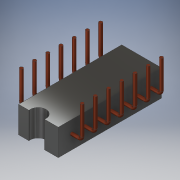
# Autodesk Inventor part: dip7
Saved by Autodesk Inventor 2019 (Build 230136000, 136)
## iProperties
Created: 2020-05-08
Part Number: dip7
Material: Silicon Nitride
Document SubType Name: Modeling
Designer: darkl
Density: 3.18 g/cm^3
Appearance: Chrome - Polished Black
Author: darkl
Autodesk Inventor part; units mm, degrees
ref_plane "YZ Plane" through (0, 0, 0) normal (1, 0, 0) x (0, 1, 0)
ref_plane "XZ Plane" through (0, 0, 0) normal (0, 1, 0) x (-1, 0, 0)
ref_plane "XY Plane" through (0, 0, 0) normal (0, 0, 1) x (1, 0, 0)
sketch "Sketch1" plane through (0, 0, 0) normal (0, 1, 0) x (-1, 0, 0)
  line L0 (4.5856, 19.0159) -> (4.5856, -0.4841)
  line L1 (4.5856, -0.4841) -> (-2.9144, -0.4841)
  line L2 (-2.9144, -0.4841) -> (-2.9144, 19.0159)
  line L3 (-2.9144, 19.0159) -> (4.5856, 19.0159)
  point P0 (0, 0)
  dimension "d0" = 19.5
  dimension "d1" = 7.5
  dimension "d2" = 19.5
  constraints: 8 end point, 2 perpendicular, 1 vertical
  measures "d0" distance of L0.start L0.end
  measures "d1" distance of L0.end L1.end
  measures "d2" distance of L1.end L2.end
extrude "Extrusion1" add sketch "Sketch1" along normal blind 5
sketch "Sketch2" plane through (2.9144, 0, 19.0159) normal (1, 0, 0) x (0, 0, -1)
  circle A0 centre (17.518, 2.6919) radius 0.3
  point P0 (19.0159, 0)
  dimension "d9" = 0.6
  constraints: 1 centre point
  measures "d9" diameter of A0
sketch3d "3D Sketch2"
  line L0 (2.9144, 2.6919, 1.4979) -> (4.3144, 2.6919, 1.4979)
  arc A0 (4.3144, 2.6919, 1.4979) -> (4.9144, 3.2919, 1.4979) centre (4.3144, 3.2919, 1.4979) ccw
  line L1 (4.9144, 3.2919, 1.4979) -> (4.9144, 8.6919, 1.4979)
  dimension "d10" = 2
  dimension "d11" = 6
  dimension "d12" = 0.6
sweep "Sweep1" add profiles "Sketch2" path "3D Sketch2"
sketch "Sketch4" plane through (2.9144, 0, 19.0159) normal (1, 0, 0) x (0, 0, -1)
  circle A0 centre (17.518, 2.6919) radius 0.3 projected
  line L0 (17.518, 2.6919) -> (15.018, 2.6919)
  circle A1 centre (15.018, 2.6919) radius 0.3
  point P0 (19.0159, 0)
  dimension "d15" = 2.5
  dimension "d16" = 0.6
  constraints: 2 end point, 1 centre point, 1 coincident, 1 horizontal
  measures "d15" distance of L0.start L0.end
  measures "d16" diameter of A1
sketch3d "3D Sketch3"
  line L0 (2.9144, 2.6919, 3.9979) -> (4.3144, 2.6919, 3.9979)
  arc A0 (4.3144, 2.6919, 3.9979) -> (4.9144, 3.2919, 3.9979) centre (4.3144, 3.2919, 3.9979) ccw
  line L1 (4.9144, 3.2919, 3.9979) -> (4.9144, 8.6919, 3.9979)
  dimension "d17" = 2
  dimension "d18" = 6
  dimension "d19" = 0.6
sweep "Sweep2" add profiles "Sketch4" path "3D Sketch3" contours A1
sketch "Sketch5" plane through (2.9144, 0, 19.0159) normal (1, 0, 0) x (0, 0, -1)
  circle A0 centre (15.018, 2.6919) radius 0.3 projected
  line L0 (15.018, 2.6919) -> (12.518, 2.6919)
  circle A1 centre (12.518, 2.6919) radius 0.3
  point P0 (19.0159, 0)
  dimension "d22" = 2.5
  dimension "d23" = 0.6
  constraints: 2 end point, 1 centre point, 1 coincident, 1 horizontal
  measures "d22" distance of L0.start L0.end
  measures "d23" diameter of A1
sketch3d "3D Sketch4"
  line L0 (2.9144, 2.6919, 6.4979) -> (4.3144, 2.6919, 6.4979)
  arc A0 (4.3144, 2.6919, 6.4979) -> (4.9144, 3.2919, 6.4979) centre (4.3144, 3.2919, 6.4979) ccw
  line L1 (4.9144, 3.2919, 6.4979) -> (4.9144, 8.6919, 6.4979)
  dimension "d24" = 2
  dimension "d25" = 6
  dimension "d26" = 0.6
sweep "Sweep3" add profiles "Sketch5" path "3D Sketch4" contours A1
sketch "Sketch6" plane through (2.9144, 0, 19.0159) normal (1, 0, 0) x (0, 0, -1)
  circle A0 centre (12.518, 2.6919) radius 0.3 projected
  line L0 (12.518, 2.6919) -> (10.018, 2.6919)
  circle A1 centre (10.018, 2.6919) radius 0.3
  line L1 (10.018, 2.6919) -> (7.518, 2.6919)
  circle A2 centre (7.518, 2.6919) radius 0.3
  line L2 (7.518, 2.6919) -> (5.018, 2.6919)
  circle A3 centre (5.018, 2.6919) radius 0.3
  line L3 (5.018, 2.6919) -> (2.518, 2.6919)
  circle A4 centre (2.518, 2.6919) radius 0.3
  point P0 (19.0159, 0)
  dimension "d29" = 2.5
  dimension "d30" = 0.6
  dimension "d31" = 2.5
  dimension "d32" = 0.6
  dimension "d33" = 2.5
  dimension "d34" = 0.6
  dimension "d35" = 2.5
  dimension "d36" = 0.6
  constraints: 8 end point, 4 centre point, 4 coincident, 3 horizontal, 1 point on line
  measures "d29" distance of L0.start L0.end
  measures "d30" diameter of A1
  measures "d31" distance of L1.start L1.end
  measures "d32" diameter of A2
  measures "d33" distance of L2.start L2.end
  measures "d34" diameter of A3
  measures "d35" distance of L3.start L3.end
  measures "d36" diameter of A4
sketch3d "3D Sketch5"
  line L0 (2.9144, 2.6919, 8.9979) -> (4.3144, 2.6919, 8.9979)
  arc A0 (4.3144, 2.6919, 8.9979) -> (4.9144, 3.2919, 8.9979) centre (4.3144, 3.2919, 8.9979) ccw
  line L1 (4.9144, 3.2919, 8.9979) -> (4.9144, 8.6919, 8.9979)
  dimension "d37" = 2
  dimension "d38" = 6
  dimension "d39" = 0.6
sweep "Sweep4" add profiles "Sketch6" path "3D Sketch5" contours A1 L1 L0 | L0 L1 A1
sketch "Sketch7" plane through (2.9144, 0, 19.0159) normal (1, 0, 0) x (0, 0, -1)
  circle A0 centre (10.018, 2.6919) radius 0.3 projected
  line L0 (10.018, 2.6919) -> (7.518, 2.6919)
  circle A1 centre (7.518, 2.6919) radius 0.3
  point P0 (19.0159, 0)
  dimension "d42" = 2.5
  dimension "d43" = 0.6
  constraints: 2 end point, 1 centre point, 1 coincident, 1 horizontal
  measures "d42" distance of L0.start L0.end
  measures "d43" diameter of A1
sketch3d "3D Sketch7"
  line L0 (2.9144, 2.6919, 11.4979) -> (4.3144, 2.6919, 11.4979)
  arc A0 (4.3144, 2.6919, 11.4979) -> (4.9144, 3.2919, 11.4979) centre (4.3144, 3.2919, 11.4979) ccw
  line L1 (4.9144, 3.2919, 11.4979) -> (4.9144, 8.6919, 11.4979)
  dimension "d44" = 2
  dimension "d45" = 6
  dimension "d46" = 0.6
sweep "Sweep5" add profiles "Sketch7" path "3D Sketch7" contours A1
sketch "Sketch8" plane through (2.9144, 0, 19.0159) normal (1, 0, 0) x (0, 0, -1)
  circle A0 centre (7.518, 2.6919) radius 0.3 projected
  line L0 (7.518, 2.6919) -> (5.018, 2.6919)
  circle A1 centre (5.018, 2.6919) radius 0.3
  point P0 (19.0159, 0)
  dimension "d49" = 2.5
  dimension "d50" = 0.6
  constraints: 2 end point, 1 centre point, 1 coincident, 1 horizontal
  measures "d49" distance of L0.start L0.end
  measures "d50" diameter of A1
sketch3d "3D Sketch9"
  line L0 (2.9144, 2.6919, 13.9979) -> (4.3144, 2.6919, 13.9979)
  arc A0 (4.3144, 2.6919, 13.9979) -> (4.9144, 3.2919, 13.9979) centre (4.3144, 3.2919, 13.9979) ccw
  line L1 (4.9144, 3.2919, 13.9979) -> (4.9144, 8.6919, 13.9979)
  dimension "d51" = 2
  dimension "d52" = 6
  dimension "d53" = 0.6
sweep "Sweep6" add profiles "Sketch8" path "3D Sketch9" contours A1
sketch "Sketch9" plane through (2.9144, 0, 19.0159) normal (1, 0, 0) x (0, 0, -1)
  circle A0 centre (5.018, 2.6919) radius 0.3 projected
  line L0 (5.018, 2.6919) -> (2.518, 2.6919)
  circle A1 centre (2.518, 2.6919) radius 0.3
  point P0 (19.0159, 0)
  dimension "d56" = 2.5
  dimension "d57" = 0.6
  constraints: 2 end point, 1 centre point, 1 coincident, 1 horizontal
  measures "d56" distance of L0.start L0.end
  measures "d57" diameter of A1
sketch3d "3D Sketch10"
  line L0 (2.9144, 2.6919, 16.4979) -> (4.3144, 2.6919, 16.4979)
  arc A0 (4.3144, 2.6919, 16.4979) -> (4.9144, 3.2919, 16.4979) centre (4.3144, 3.2919, 16.4979) ccw
  line L1 (4.9144, 3.2919, 16.4979) -> (4.9144, 8.6919, 16.4979)
  dimension "d58" = 2
  dimension "d59" = 6
  dimension "d60" = 0.6
sweep "Sweep7" add profiles "Sketch9" path "3D Sketch10" contours A1
sketch "Sketch11" plane through (-4.5856, 0, -0.4841) normal (-1, 0, 0) x (0, 0, 1)
  circle A0 centre (1.982, 2.6919) radius 0.3 projected
  circle A1 centre (1.982, 2.6919) radius 0.3
  point P0 (0.4841, 0)
  dimension "d64" = 0.6
  constraints: 1 centre point, 1 coincident
  measures "d64" diameter of A1
sketch3d "3D Sketch12"
  line L0 (-4.5856, 2.6919, 1.4979) -> (-5.9856, 2.6919, 1.4979)
  arc A0 (-5.9856, 2.6919, 1.4979) -> (-6.5856, 3.2919, 1.4979) centre (-5.9856, 3.2919, 1.4979) ccw
  line L1 (-6.5856, 3.2919, 1.4979) -> (-6.5856, 8.6919, 1.4979)
  dimension "d65" = 2
  dimension "d66" = 6
  dimension "d67" = 0.6
sweep "Sweep8" add profiles "Sketch11" path "3D Sketch12"
sketch "Sketch12" plane through (-4.5856, 0, -0.4841) normal (-1, 0, 0) x (0, 0, 1)
  circle A0 centre (1.982, 2.6919) radius 0.3 projected
  line L0 (1.982, 2.6919) -> (4.482, 2.6919)
  circle A1 centre (4.482, 2.6919) radius 0.3 projected
  circle A2 centre (4.482, 2.6919) radius 0.3
  point P0 (0.4841, 0)
  dimension "d70" = 2.5
  dimension "d71" = 0.6
  constraints: 2 end point, 1 centre point, 1 coincident, 1 horizontal
  measures "d70" distance of L0.start L0.end
  measures "d71" diameter of A2
sketch3d "3D Sketch13"
  line L0 (-4.5856, 2.6919, 3.9979) -> (-5.9856, 2.6919, 3.9979)
  arc A0 (-5.9856, 2.6919, 3.9979) -> (-6.5856, 3.2919, 3.9979) centre (-5.9856, 3.2919, 3.9979) ccw
  line L1 (-6.5856, 3.2919, 3.9979) -> (-6.5856, 8.6919, 3.9979)
  dimension "d72" = 2
  dimension "d73" = 6
  dimension "d74" = 0.6
sweep "Sweep9" add profiles "Sketch12" path "3D Sketch13" contours A1
sketch "Sketch13" plane through (-4.5856, 0, -0.4841) normal (-1, 0, 0) x (0, 0, 1)
  circle A0 centre (4.482, 2.6919) radius 0.3 projected
  line L0 (4.482, 2.6919) -> (6.982, 2.6919)
  circle A1 centre (6.982, 2.6919) radius 0.3
  point P0 (0.4841, 0)
  dimension "d77" = 2.5
  dimension "d78" = 0.6
  constraints: 2 end point, 1 centre point, 1 coincident, 1 horizontal
  measures "d77" distance of L0.start L0.end
  measures "d78" diameter of A1
sketch3d "3D Sketch14"
  line L0 (-4.5856, 2.6919, 6.4979) -> (-5.9856, 2.6919, 6.4979)
  arc A0 (-5.9856, 2.6919, 6.4979) -> (-6.5856, 3.2919, 6.4979) centre (-5.9856, 3.2919, 6.4979) ccw
  line L1 (-6.5856, 3.2919, 6.4979) -> (-6.5856, 8.6919, 6.4979)
  dimension "d79" = 2
  dimension "d80" = 6
  dimension "d81" = 0.6
sweep "Sweep10" add profiles "Sketch13" path "3D Sketch14" contours A1
sketch "Sketch14" plane through (-4.5856, 0, -0.4841) normal (-1, 0, 0) x (0, 0, 1)
  circle A0 centre (6.982, 2.6919) radius 0.3 projected
  circle A1 centre (9.482, 2.6919) radius 0.3 projected
  line L0 (6.982, 2.6919) -> (9.482, 2.6919)
  circle A2 centre (9.482, 2.6919) radius 0.3
  point P0 (0.4841, 0)
  dimension "d84" = 2.5
  dimension "d85" = 0.6
  constraints: 2 end point, 1 centre point, 1 coincident, 1 horizontal
  measures "d84" distance of L0.start L0.end
  measures "d85" diameter of A2
sketch3d "3D Sketch15"
  line L0 (-4.5856, 2.6919, 8.9979) -> (-5.9856, 2.6919, 8.9979)
  arc A0 (-5.9856, 2.6919, 8.9979) -> (-6.5856, 3.2919, 8.9979) centre (-5.9856, 3.2919, 8.9979) ccw
  line L1 (-6.5856, 3.2919, 8.9979) -> (-6.5856, 8.6919, 8.9979)
  dimension "d86" = 2
  dimension "d87" = 6
  dimension "d88" = 0.6
sweep "Sweep11" add profiles "Sketch14" path "3D Sketch15" contours A1
sketch "Sketch15" plane through (-4.5856, 0, -0.4841) normal (-1, 0, 0) x (0, 0, 1)
  circle A0 centre (9.482, 2.6919) radius 0.3 projected
  circle A1 centre (11.982, 2.6919) radius 0.3 projected
  line L0 (9.482, 2.6919) -> (11.982, 2.6919)
  circle A2 centre (11.982, 2.6919) radius 0.3
  point P0 (0.4841, 0)
  dimension "d91" = 2.5
  dimension "d92" = 0.6
  constraints: 2 end point, 1 centre point, 1 coincident, 1 horizontal
  measures "d91" distance of L0.start L0.end
  measures "d92" diameter of A2
sketch3d "3D Sketch17"
  line L0 (-4.5856, 2.6919, 11.4979) -> (-5.9856, 2.6919, 11.4979)
  arc A0 (-5.9856, 2.6919, 11.4979) -> (-6.5856, 3.2919, 11.4979) centre (-5.9856, 3.2919, 11.4979) ccw
  line L1 (-6.5856, 3.2919, 11.4979) -> (-6.5856, 8.6919, 11.4979)
  dimension "d93" = 2
  dimension "d94" = 6
  dimension "d95" = 0.6
sweep "Sweep12" add profiles "Sketch15" path "3D Sketch17" contours A1
sketch "Sketch16" plane through (-4.5856, 0, -0.4841) normal (-1, 0, 0) x (0, 0, 1)
  circle A0 centre (11.982, 2.6919) radius 0.3 projected
  line L0 (11.982, 2.6919) -> (14.482, 2.6919)
  circle A1 centre (14.482, 2.6919) radius 0.3 projected
  circle A2 centre (14.482, 2.6919) radius 0.3
  point P0 (0.4841, 0)
  dimension "d98" = 2.5
  dimension "d99" = 0.6
  constraints: 2 end point, 1 centre point, 1 coincident, 1 horizontal
  measures "d98" distance of L0.start L0.end
  measures "d99" diameter of A2
sketch3d "3D Sketch18"
  line L0 (-4.5856, 2.6919, 13.9979) -> (-5.9856, 2.6919, 13.9979)
  arc A0 (-5.9856, 2.6919, 13.9979) -> (-6.5856, 3.2919, 13.9979) centre (-5.9856, 3.2919, 13.9979) ccw
  line L1 (-6.5856, 3.2919, 13.9979) -> (-6.5856, 8.6919, 13.9979)
  dimension "d100" = 2
  dimension "d101" = 6
  dimension "d102" = 0.6
sweep "Sweep13" add profiles "Sketch16" path "3D Sketch18" contours A1
sketch "Sketch17" plane through (-4.5856, 0, -0.4841) normal (-1, 0, 0) x (0, 0, 1)
  circle A0 centre (14.482, 2.6919) radius 0.3 projected
  line L0 (14.482, 2.6919) -> (16.982, 2.6919)
  circle A1 centre (16.982, 2.6919) radius 0.3 projected
  circle A2 centre (16.982, 2.6919) radius 0.3
  point P0 (0.4841, 0)
  dimension "d105" = 2.5
  dimension "d106" = 0.6
  constraints: 2 end point, 1 centre point, 1 coincident, 1 horizontal
  measures "d105" distance of L0.start L0.end
  measures "d106" diameter of A2
sketch3d "3D Sketch19"
  line L0 (-4.5856, 2.6919, 16.4979) -> (-5.9856, 2.6919, 16.4979)
  arc A0 (-5.9856, 2.6919, 16.4979) -> (-6.5856, 3.2919, 16.4979) centre (-5.9856, 3.2919, 16.4979) ccw
  line L1 (-6.5856, 3.2919, 16.4979) -> (-6.5856, 8.6919, 16.4979)
  dimension "d107" = 2
  dimension "d108" = 6
  dimension "d109" = 0.6
sweep "Sweep14" add profiles "Sketch17" path "3D Sketch19" contours A1
sketch "Sketch18" plane through (0, 0, 0) normal (0, -1, 0) x (1, 0, 0)
  point P0 (0, 0)
  point P1 (-1.1633, 18.7506)
hole "Hole1" at (-1.1633, 0, 18.7506) direction (0, 1, 0) diameter 3 depth 8 tip angle 118
body "Solid1"
